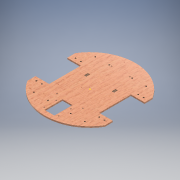
# Autodesk Inventor part: 底盤
Saved by Autodesk Inventor 2017 (Build 210142000, 142)
## iProperties
Created: 2019-10-03
Part Number: 底盤
Material: Generic
Document SubType Name: Modeling
Designer: User
Density: 1 g/cm^3
Appearance: Weld - Aluminum
Author: User
Autodesk Inventor part; units mm, degrees
ref_plane "YZ Plane" through (0, 0, 0) normal (1, 0, 0) x (0, 1, 0)
ref_plane "XZ Plane" through (0, 0, 0) normal (0, 1, 0) x (-1, 0, 0)
sketch "Sketch1" plane through (0, 0, 0) normal (0, 0, 1) x (1, 0, 0)
  line L0 (85, -35) -> (55, -35)
  line L1 (55, -35) -> (55, 35)
  line L2 (55, 35) -> (85, 35)
  line L3 (85, 35) -> (85, -35)
  line L4 (85, -35) -> (55, 35) construction
  line L5 (55, -35) -> (85, 35) construction
  line L6 (-85, -35) -> (-55, -35)
  line L7 (-55, -35) -> (-55, 35)
  line L8 (-55, 35) -> (-85, 35)
  line L9 (-85, 35) -> (-85, -35)
  line L10 (-85, 35) -> (-85, 52.6783)
  line L11 (-85, -35) -> (-85, -52.6783)
  line L12 (85, 35) -> (85, 52.6783)
  line L13 (85, -35) -> (85, -52.6783)
  arc A0 (-85, -52.6783) -> (85, -52.6783) centre (0, 0) ccw
  arc A1 (85, 52.6783) -> (-85, 52.6783) centre (0, 0) ccw
  point P0 (70, 0)
  dimension "d6" = 30
  dimension "d7" = 70
  dimension "d155" = 100
  constraints: 28 end point, 4 point on circle, 3 parallel, 2 centre point, 2 midpoint, 2 point on line, 1 coincident, 1 horizontal, 1 perpendicular, 1 vertical
  measures "d6" distance of L1.end L2.end
  measures "d7" distance of L0.end L1.end
  measures "d155" radius of A1
extrude "Extrusion2" add sketch "Sketch1" along normal blind 3 contours L13 A0 L11 L6 L7 L8 L10 A1 L12 L2 L1 L0
sketch "Sketch3" plane through (0, 0, 0) normal (1, 0, 0) x (0, 1, 0)
  point P0 (0, 0)
ref_plane "Work Plane1" through (-33, -35, 0) normal (-1, 0, 0) x (0, 0, 1)
sketch "Sketch21" plane through (0, 0, 3) normal (0, 0, 1) x (1, 0, 0)
  line L0 (11, -59.3932) -> (11, -49.3932)
  line L1 (11, -49.3932) -> (-11, -49.3932)
  line L2 (-11, -49.3932) -> (11, -49.3932)
  line L3 (11, -49.3932) -> (11, -89.3932)
  line L4 (-11, -49.3932) -> (-11, -89.3932)
  line L5 (-11, -89.3932) -> (11, -89.3932)
  point P0 (0, 0)
  dimension "d149" = 40
  constraints: 12 end point, 2 perpendicular, 1 horizontal
  measures "d149" distance of L1.end L4.end
sketch "Sketch31" plane through (0, 0, 3) normal (0, 0, 1) x (1, 0, 0)
  circle A0 centre (-56, -67.5) radius 1.5 projected
  circle A1 centre (-56, -67.5) radius 1.5
  circle A2 centre (-25, -67.5) radius 1.5 projected
  circle A3 centre (-25, -67.5) radius 1.5
  point P0 (0, 0)
  dimension "d117" = 3
  dimension "d118" = 3
  constraints: 2 centre point, 2 coincident
  measures "d117" diameter of A1
  measures "d118" diameter of A3
extrude "Extrusion30" cut sketch "Sketch31" against normal up to next
mirror "Mirror19" about plane through (0, 0, 0) normal (0, 1, 0) of "Extrusion30"
mirror "Mirror20" about plane through (0, 0, 0) normal (1, 0, 0) of "Extrusion30", "Mirror19"
sketch "Sketch32" plane through (0, 0, 3) normal (0, 0, 1) x (1, 0, 0)
  line L0 (-33, 28) -> (-28, 28) projected
  line L1 (-28, 28) -> (-28, 20) projected
  line L2 (-33, 28) -> (-28, 28)
  line L3 (-28, 28) -> (-28, 20)
  line L4 (-28, 20) -> (-33, 20)
  line L5 (-33, 20) -> (-33, 28)
  line L6 (33, 28) -> (28, 28) projected
  line L7 (28, 28) -> (33, 28)
  line L8 (33, 28) -> (33, 20)
  line L9 (33, 20) -> (28, 20)
  line L10 (28, 20) -> (28, 28)
  point P0 (0, 0)
  constraints: 16 end point, 4 parallel, 2 horizontal, 2 perpendicular
extrude "Extrusion31" cut sketch "Sketch32" against normal blind 1
sketch "Sketch33" plane through (0, 0, 0) normal (0, 0, -1) x (-1, 0, 0)
  line L0 (-60, 40) -> (-78, 40)
  line L1 (-78, 40) -> (-78, 46)
  line L2 (-78, 46) -> (-60, 46)
  line L3 (-60, 46) -> (-60, 40)
  point P0 (0, 0)
  dimension "d123" = 18
  dimension "d124" = 6
  constraints: 8 end point, 2 parallel, 1 horizontal, 1 perpendicular
  measures "d123" distance of L1.end L2.end
  measures "d124" distance of L0.end L1.end
extrude "Extrusion32" cut sketch "Sketch33" against normal blind 1
mirror "Mirror21" about plane through (0, 0, 0) normal (1, 0, 0) of "Extrusion32"
mirror "Mirror22" about plane through (0, 0, 0) normal (0, 1, 0) of "Extrusion32", "Mirror21"
sketch "Sketch34" plane through (0, 0, 1) normal (0, 0, -1) x (-1, 0, 0)
  circle A0 centre (-75, 43) radius 1.5
  circle A1 centre (-63, 43) radius 1.5
  point P0 (0, 0)
  dimension "d127" = 3
  dimension "d128" = 3
  constraints: 2 centre point
  measures "d127" diameter of A0
  measures "d128" diameter of A1
extrude "Extrusion33" cut sketch "Sketch34" against normal up to next
mirror "Mirror23" about plane through (0, 0, 0) normal (1, 0, 0) of "Extrusion33"
mirror "Mirror24" about plane through (0, 0, 0) normal (0, 1, 0) of "Extrusion33", "Mirror23"
sketch "Sketch35" plane through (0, 0, 3) normal (0, 0, 1) x (1, 0, 0)
  point P0 (0, 0)
extrude "Extrusion35" cut sketch "Sketch21" against normal up to next
sketch "Sketch37" plane through (0, 0, 3) normal (0, 0, 1) x (1, 0, 0)
  line L0 (0, -58.4467) -> (16, -58.4467)
  circle A0 centre (16, -58.4467) radius 1.5
  circle A1 centre (16, -85) radius 1.5
  point P0 (0, 0)
  dimension "d137" = 16
  dimension "d138" = 3
  dimension "d139" = 3
  constraints: 2 centre point, 2 end point, 1 coincident, 1 horizontal
  measures "d137" distance of L0.start L0.end
  measures "d138" diameter of A0
  measures "d139" diameter of A1
extrude "Extrusion36" cut sketch "Sketch37" against normal up to next
mirror "Mirror25" about plane through (0, 0, 0) normal (1, 0, 0) of "Extrusion36"
sketch "Sketch38" plane through (0, 0, 3) normal (0, 0, 1) x (1, 0, 0)
  circle A0 centre (-25, -67.5) radius 1.5 projected
  line L0 (-25, -67.5) -> (11, -67.5) construction
  circle A1 centre (-56, 67.5) radius 1.5 projected
  circle A2 centre (-20, 67.5) radius 1.5
  circle A3 centre (-56, -67.5) radius 1.5 projected
  line L1 (-56, -67.5) -> (-20, -67.5) construction
  circle A4 centre (-28.4224, -44.3596) radius 1.5
  point P0 (0, 0)
  dimension "d146" = 3
  dimension "d152" = 3
  constraints: 4 end point, 2 centre point, 2 horizontal
  measures "d146" diameter of A2
  measures "d152" diameter of A4
extrude "Extrusion38" cut sketch "Sketch38" against normal up to next contours A2 | A4
mirror "Mirror27" about plane through (0, 0, 0) normal (1, 0, 0) of "Extrusion38"
body "Solid2"
